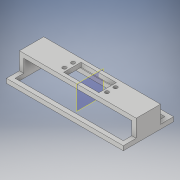
# Autodesk Inventor part: МД.001.1002 - Направляющие
Saved by Autodesk Inventor 2019 (Build 230136000, 136)
## iProperties
Created: 2019-12-30
Part Number: МД.001.1002 - Направляющие
Material: Типовые
Document SubType Name: Modeling
Designer: Петров Иван
Density: 1 g/cm^3
Appearance: По умолчанию
Author: Петров Иван
Autodesk Inventor part; units mm, degrees
ref_plane "YZ Plane" through (0, 0, 0) normal (1, 0, 0) x (0, 1, 0)
ref_plane "XZ Plane" through (0, 0, 0) normal (0, 1, 0) x (-1, 0, 0)
ref_plane "XY Plane" through (0, 0, 0) normal (0, 0, 1) x (1, 0, 0)
sketch "Эскиз1" plane through (0, 0, 0) normal (0, 1, 0) x (-1, 0, 0)
  line L0 (-10, -10) -> (-10, 10)
  line L1 (-10, 10) -> (-16, 10)
  arc A0 (-16, 10) -> (-17, 9) centre (-16, 9) ccw
  line L2 (-17, 9) -> (-17, 6.15)
  line L3 (-17, 6.15) -> (-15.934, 6.15)
  arc A1 (-15.934, 3.75) -> (-15.934, 6.15) centre (-14.15, 4.95) ccw
  line L4 (-15.934, 3.75) -> (-17, 3.75)
  line L5 (-17, 3.75) -> (-17, -3.75)
  line L6 (-17, -3.75) -> (-15.934, -3.75)
  arc A2 (-15.934, -6.15) -> (-15.934, -3.75) centre (-14.15, -4.95) ccw
  line L7 (-15.934, -6.15) -> (-17, -6.15)
  line L8 (-17, -6.15) -> (-17, -9)
  arc A3 (-17, -9) -> (-16, -10) centre (-16, -9) ccw
  line L9 (-16, -10) -> (-10, -10)
  line L10 (37.7, -3.75) -> (36.634, -3.75)
  line L11 (37.7, 3.75) -> (37.7, -3.75)
  line L12 (36.634, 3.75) -> (37.7, 3.75)
  arc A4 (36.634, 6.15) -> (36.634, 3.75) centre (34.85, 4.95) ccw
  line L13 (37.7, 6.15) -> (36.634, 6.15)
  line L14 (37.7, 9) -> (37.7, 6.15)
  arc A5 (37.7, 9) -> (36.7, 10) centre (36.7, 9) ccw
  line L15 (30.7, 10) -> (36.7, 10)
  line L16 (30.7, -10) -> (30.7, 10)
  line L17 (36.7, -10) -> (30.7, -10)
  arc A6 (36.7, -10) -> (37.7, -9) centre (36.7, -9) ccw
  line L18 (37.7, -6.15) -> (37.7, -9)
  line L19 (36.634, -6.15) -> (37.7, -6.15)
  arc A7 (36.634, -3.75) -> (36.634, -6.15) centre (34.85, -4.95) ccw
  line L20 (-10, 10) -> (30.7, 10)
  line L21 (30.7, -10) -> (-10, -10)
  line L22 (-10, -10) -> (-10, 10)
  circle A8 centre (0, 0) radius 1.25
  circle A9 centre (0, 0) radius 3.4957
  circle A10 centre (0, 0) radius 2.6787
  circle A11 centre (0, 0) radius 5.4
  line L23 (37.7, 6.15) -> (37.7, 3.75)
  line L24 (37.7, -3.75) -> (37.7, -6.15)
  line L25 (37.7, 3.75) -> (37.7, 0.5)
  line L26 (-17, 3.75) -> (-17, -3.75)
  line L27 (-17, 6.15) -> (-17, 3.75)
  line L28 (-17, 3.75) -> (-17, -3.75)
  line L29 (-17, -3.75) -> (-17, -6.15)
  circle A12 centre (-14.15, 4.95) radius 2.15
  circle A13 centre (-14.15, -4.95) radius 2.15
  arc A14 (36.634, -3.75) -> (36.634, -6.15) centre (34.85, -4.95) ccw
  circle A15 centre (34.85, -4.95) radius 2.15
  circle A16 centre (34.85, 4.95) radius 2.15
  line L30 (37.7, 9) -> (37.7, 14)
  line L31 (37.7, 14) -> (-17, 14)
  line L32 (-17, 14) -> (-17, 9)
  line L33 (37.7, -9) -> (37.7, -14)
  line L34 (37.7, -14) -> (-17, -14)
  line L35 (-17, -14) -> (-17, -9)
  point P0 (10.35, -10)
  dimension "d0" = 5
  dimension "d1" = 5
  constraints: 72 end point, 18 point on circle, 16 centre point, 4 coincident, 4 collinear, 4 point on line, 2 concentric, 2 perpendicular, 2 vertical, 3 other
  measures "d0" distance of L14.start L30.end
  measures "d1" distance of L18.end L33.end
extrude "Выдавливание1" add sketch "Эскиз1" along normal blind 5 contours L9 A3 L8 L7 A2 L6 L5 L4 A1 L3 L2 A0 L1 L0 | L21 L17 A6 L33 L34 L35 A3 L9 | L1 A0 L32 L31 L30 A5 L15 L20 | L16 L15 A5 L14 L13 A4 L12 L11 L10 A7 L19 L18 A6 L17 | L29 L6 A13 L7 | L3 A12 L4 L27 | L19 A15 L10 L24 | L23 L12 A16 L13
sketch "Эскиз2" plane through (17, 0, 14) normal (1, 0, 0) x (0, 0, -1)
  line L0 (0, 5) -> (28, 5) projected
  line L1 (0, 0) -> (28, 0) projected
  line L2 (0, 5) -> (28, 5)
  line L3 (28, 5) -> (28, 0)
  line L4 (28, 0) -> (0, 0)
  line L5 (0, 0) -> (0, 5)
  point P0 (14, 0)
  constraints: 8 end point, 2 parallel, 1 horizontal, 1 perpendicular
extrude "Выдавливание2" add sketch "Эскиз2" along normal blind 40
sketch "Эскиз3" plane through (0, 5, 0) normal (0, 1, 0) x (1, 0, 0)
  line L0 (-37.7, -14) -> (57, -14) projected
  line L1 (57, 14) -> (52, 14)
  line L2 (52, 14) -> (52, -14)
  line L3 (52, -14) -> (57, -14)
  line L4 (57, -14) -> (57, 14)
  point P0 (0, 0)
  dimension "d6" = 5
  constraints: 8 end point, 2 parallel, 1 horizontal, 1 perpendicular, 1 point on line
  measures "d6" distance of L3.end L2.end
extrude "Выдавливание3" add sketch "Эскиз3" against normal blind 25
ref_plane "РабПлоскость1" through (-10.35, 0, 10) normal (-1, 0, 0) x (0, 0, 1)
sketch "Эскиз4" plane through (57, 0, 14) normal (1, 0, 0) x (0, 0, -1)
  line L0 (28, -20) -> (43, -20)
  line L1 (43, -20) -> (43, -15)
  line L2 (43, -15) -> (28, -15)
  line L3 (28, -15) -> (28, -20)
  line L4 (0, -20) -> (-15, -20)
  line L5 (-15, -20) -> (-15, -15)
  line L6 (-15, -15) -> (0, -15)
  line L7 (0, -15) -> (0, -20)
  point P0 (14, 0)
  dimension "d9" = 15
  dimension "d10" = 15
  dimension "d11" = 5
  dimension "d12" = 5
  constraints: 16 end point, 4 parallel, 2 horizontal, 2 perpendicular
  measures "d9" distance of L2.end L1.end
  measures "d10" distance of L5.end L6.end
  measures "d11" distance of L4.end L5.end
  measures "d12" distance of L0.end L1.end
extrude "Выдавливание4" add sketch "Эскиз4" against normal blind 5
sketch "Эскиз5" plane through (52, 0, -14) normal (-1, 0, 0) x (0, 0, 1)
  line L0 (43, -20) -> (-15, -20) projected
  line L1 (43, -20) -> (38, -20)
  line L2 (38, -20) -> (38, -15)
  line L3 (38, -15) -> (43, -15)
  line L4 (43, -15) -> (43, -20)
  line L5 (-15, -15) -> (-15, -20) projected
  line L6 (-15, -15) -> (-10, -15)
  line L7 (-10, -15) -> (-10, -20)
  line L8 (-10, -20) -> (-15, -20)
  line L9 (-15, -20) -> (-15, -15)
  point P0 (14, 0)
  dimension "d15" = 5
  dimension "d16" = 5
  dimension "d17" = 5
  dimension "d18" = 5
  constraints: 16 end point, 4 parallel, 2 horizontal, 2 perpendicular
  measures "d15" distance of L2.end L3.end
  measures "d16" distance of L1.end L2.end
  measures "d17" distance of L7.end L8.end
  measures "d18" distance of L6.end L7.end
extrude "Выдавливание5" add sketch "Эскиз5" along normal up to surface (62.35 mm away)
mirror "Зеркальное отражение2" about plane through (-10.35, 0, 10) normal (-1, 0, 0) of "Выдавливание3", "Выдавливание4", "Выдавливание5", "Выдавливание2"
